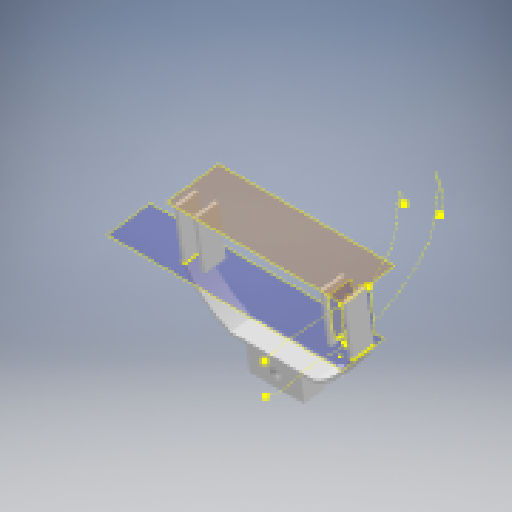
# Autodesk Inventor part: imu_mount
Saved by Autodesk Inventor 2024 (Build 280153000, 153)
## iProperties
Created: 2025-01-05
Part Number: imu_mount
Material: Generic
Document SubType Name: Modeling
Designer: Alex
Density: 1 g/cm^3
Appearance: Default
Author: Alex
Autodesk Inventor part; units mm, degrees
ref_plane "YZ Plane" through (0, 0, 0) normal (1, 0, 0) x (0, 1, 0)
ref_plane "XZ Plane" through (0, 0, 0) normal (0, 1, 0) x (-1, 0, 0)
ref_plane "XY Plane" through (0, 0, 0) normal (0, 0, 1) x (1, 0, 0)
sketch "Sketch1" plane through (0, 0, 0) normal (1, 0, 0) x (0, 1, 0)
  spline S0 degree 3 poles (-12.7596, 69.1102) (-15.2298, 61.5354) (-16.003, 54.7493) (-14.7341, 46.512) (-13.9585, 44.5403) (-12.6997, 40.1512) (-11.8689, 37.886) (-10.5675, 32.6221) (-10.0341, 29.5076) (-9.2498, 23.4956) (-9.1586, 20.4828) (-8.7362, 14.9457) (-8.298, 12.4468) (-8.4378, 7.0305) (-9.5013, 4.1287) (-9.4732, -0.7666) (-9.0812, -2.8089) (-8.7088, -6.0813) (-8.5625, -7.3217) (-8.4075, -8.5547) knots 0 0 0 0 0.241973 0.241973 0.332352 0.332352 0.424089 0.424089 0.541798 0.541798 0.658072 0.658072 0.76087 0.76087 0.872069 0.872069 0.951758 0.951758 1 1 1 1 construction
  spline S1 degree 3 poles (-8.4075, -8.5547) (-8.309, -9.3389) (-8.207, -10.12) (-7.7153, -13.7099) (-7.2118, -16.3393) (-6.3841, -22.1405) (-6.6665, -24.8142) (-5.6218, -28.3135) knots 0 0 0 0 0.119502 0.119502 0.553846 0.553846 1 1 1 1 construction
  spline S2 degree 3 poles (-5.6218, -28.3135) (-4.1228, -33.3346) (0.624, -41.8906) (3.9625, -48.268) (4.5736, -49.3774) (8.1498, -55.2575) (12.792, -61.9002) (17.7565, -68.8098) (19.0389, -70.9296) (26.2047, -78.6536) (35.4784, -85.2147) (49.0059, -92.3069) (55.6073, -92.3063) (68.5377, -94.6562) (74.996, -95.2419) (83.2666, -94.7145) (86.6124, -93.0362) (89.415, -93.015) (89.4684, -93.7995) (89.9841, -94.339) (90.2258, -94.7218) (89.67, -94.6644) (89.4356, -94.0936) (87.2104, -94.21) (84.8902, -94.7513) (80.0382, -96.05) (76.8909, -97.5474) (70.3825, -98.6246) (66.2945, -98.5443) (60.1257, -98.0168) (58.2481, -97.7121) (54.5132, -96.7744) (53.8418, -96.5978) (53.124, -96.4018) knots 0 0 0 0 0.060463 0.060463 0.088876 0.088876 0.149034 0.149034 0.189187 0.189187 0.280144 0.280144 0.381032 0.381032 0.501928 0.501928 0.587779 0.587779 0.653298 0.653298 0.710459 0.710459 0.757232 0.757232 0.814775 0.814775 0.872532 0.872532 0.939307 0.939307 0.990036 0.990036 1 1 1 1 construction
  spline S3 degree 3 poles (29.4725, -27.9505) (29.7232, -28.7604) (30.1347, -29.057) (32.5515, -32.3248) (34.3621, -34.4691) (37.878, -38.892) (37.7974, -39.3941) (41.586, -43.4308) (43.873, -45.7682) (49.5626, -50.6314) (51.8392, -50.9545) (60.2395, -53.9595) (66.6243, -55.2783) (76.7213, -57.0347) (82.4961, -56.8836) (87.4768, -57.2216) (87.6182, -57.0776) (89.8132, -57.4611) (91.5195, -57.7058) (92.188, -58.3474) (92.2546, -58.677) (90.5785, -59.545) (88.9174, -60.1439) (85.9397, -61.0379) (84.1283, -61.4382) (81.4338, -61.8751) (80.6089, -61.9837) (79.7567, -62.0753) knots 0 0 0 0 0.04737 0.04737 0.082065 0.082065 0.155524 0.155524 0.204555 0.204555 0.315622 0.315622 0.438816 0.438816 0.586443 0.586443 0.691275 0.691275 0.771281 0.771281 0.841079 0.841079 0.898194 0.898194 0.96846 0.96846 1 1 1 1 construction
  spline S4 degree 3 poles (28.8564, -23.7777) (28.9042, -24.5022) (28.9667, -25.1696) (29.2425, -26.8854) (29.3324, -27.498) (29.4725, -27.9505) knots 0 0 0 0 0.335914 0.335914 1 1 1 1 construction
  spline S5 degree 3 poles (27.5568, -11.1594) (27.8944, -13.1016) (28.2256, -15.1008) (28.7027, -19.1945) (28.7203, -21.7171) (28.8564, -23.7777) knots 0 0 0 0 0.46171 0.46171 1 1 1 1 construction
  spline S6 degree 3 poles (26.2925, -4.4074) (26.5211, -5.6352) (26.805, -6.8301) (27.1945, -9.1012) (27.3765, -10.1222) (27.5568, -11.1594) knots 0 0 0 0 0.568778 0.568778 1 1 1 1 construction
  spline S7 degree 3 poles (16.0432, 69.6268) (18.6865, 66.183) (20.6385, 61.0286) (22.3448, 51.7367) (22.7474, 48.7933) (23.2098, 43.6518) (23.1117, 41.1975) (23.483, 35.6031) (24.0275, 32.6396) (24.3977, 26.501) (24.1107, 23.3997) (24.6444, 17.6215) (25.4306, 14.8381) (25.926, 9.3729) (25.7134, 6.8435) (25.8358, 1.9262) (25.7789, -0.3383) (26.0611, -3.0685) (26.1687, -3.7428) (26.2925, -4.4074) knots 0 0 0 0 0.257427 0.257427 0.348427 0.348427 0.440796 0.440796 0.559313 0.559313 0.676387 0.676387 0.779892 0.779892 0.891856 0.891856 0.972092 0.972092 1 1 1 1 construction
  point P0 (0, 0)
ref_plane "Work Plane1" through (0, -5.6218, -28.3135) normal (-1, 0, 0) x (0, -0.1396054, 0.9902072)
ref_plane "Work Plane2" through (5.08, -5.6218, -28.3135) normal (-1, 0, 0) x (0, -0.1396054, 0.9902072)
sketch "Sketch2" plane through (5.08, -5.6218, -28.3135) normal (-1, 0, 0) x (0, -0.1396054, 0.9902072)
  line L0 (3.8114, -6.7133) -> (24.329, -6.7133)
  line L1 (24.329, -6.7133) -> (24.329, 43.4294)
  line L2 (24.329, 43.4294) -> (3.8114, 43.4294)
  line L3 (3.8114, 43.4294) -> (3.8114, -6.7133)
  point P0 (27.2514, 9.5195)
  constraints: 8 end point, 2 parallel, 1 horizontal, 1 perpendicular
extrude "Extrusion1" add sketch "Sketch2" against normal blind 3.175
ref_plane "Work Plane3" through (-11.938, -5.6218, -28.3135) normal (-1, 0, 0) x (0, -0.1396054, 0.9902072)
sketch "Sketch3" plane through (-11.938, -5.6218, -28.3135) normal (-1, 0, 0) x (0, -0.1396054, 0.9902072)
  line L0 (24.329, -6.7133) -> (24.329, 43.4294) projected
  line L1 (24.329, 43.4294) -> (3.8114, 43.4294) projected
  line L2 (3.8114, 43.4294) -> (3.8114, -6.7133) projected
  line L3 (3.8114, -6.7133) -> (24.329, -6.7133) projected
  point P0 (27.2514, 9.5195)
extrude "Extrusion2" add sketch "Sketch3" along normal blind 3.175
sketch "Sketch4" plane through (5.08, -5.6218, -28.3135) normal (-1, 0, 0) x (0, -0.1396054, 0.9902072)
  point P0 (27.2514, 9.5195)
ref_plane "Work Plane4" through (6.6675, 33.9858, 1.8402) normal (0, 0.9902072, 0.1396054) x (0, 0.1396054, -0.9902072)
ref_plane "Work Plane5" through (8.255, -12.8015, -25.4766) normal (0, -0.9902072, -0.1396054) x (0, -0.1396054, 0.9902072)
sketch "Sketch5" plane through (8.255, -12.8015, -25.4766) normal (0, -0.9902072, -0.1396054) x (0, -0.1396054, 0.9902072)
  line L0 (0, 20.193) -> (0, 23.368) construction
  line L1 (20.5176, 20.193) -> (20.5176, 23.368) construction
  line L2 (0, 23.368) -> (0, 209.8691) construction
  line L3 (0, 143.7138) -> (20.5176, 143.7138)
  line L4 (20.5176, 143.7138) -> (20.5176, 140.5388)
  line L5 (20.5176, 140.5388) -> (0, 140.5388)
  line L6 (0, 140.5388) -> (0, 143.7138)
  line L7 (0, 162.2606) -> (20.5176, 162.2606)
  line L8 (20.5176, 162.2606) -> (20.5176, 159.0856)
  line L9 (20.5176, 159.0856) -> (0, 159.0856)
  line L10 (0, 159.0856) -> (0, 162.2606)
  point P0 (23.44, 8.255)
  dimension "d6" = 3.175
  dimension "d7" = 3.175
  constraints: 18 end point, 4 parallel, 3 point on line, 2 horizontal, 2 perpendicular, 1 vertical
  measures "d6" distance of L3.end L4.end
  measures "d7" distance of L7.end L8.end
extrude "Extrusion3" add sketch "Sketch5" against normal up to surface (50.1427 mm away)
sketch "Sketch7" plane through (8.255, -12.8015, -25.4766) normal (0, -0.9902072, -0.1396054) x (0, -0.1396054, 0.9902072)
  line L0 (0, 3.175) -> (20.5176, 3.175) projected
  line L1 (0, 3.175) -> (0, 0) projected
  line L2 (20.5176, 0) -> (0, 0) projected
  line L3 (20.5176, 3.175) -> (20.5176, 0) projected
  line L4 (0, 159.0856) -> (20.5176, 159.0856) projected
  line L5 (20.5176, 159.0856) -> (20.5176, 162.2606) projected
  line L6 (20.5176, 162.2606) -> (0, 162.2606) projected
  line L7 (0, 162.2606) -> (0, 159.0856) projected
  point P0 (23.44, 8.255)
sketch "Sketch8" plane through (-154.0056, -15.6658, -5.16) normal (0, -0.1396054, 0.9902072) x (1, 0, 0)
  line L0 (159.0856, 0) -> (159.0856, 50.1427) projected
  line L1 (159.0856, 0) -> (162.2606, 0) projected
  line L2 (162.2606, 50.1427) -> (162.2606, 0) projected
  line L3 (159.0856, 50.1427) -> (162.2606, 50.1427) projected
  line L4 (3.175, 50.1427) -> (0, 50.1427) projected
  line L5 (0, 0) -> (0, 50.1427) projected
  line L6 (3.175, 0) -> (0, 0) projected
  line L7 (3.175, 0) -> (3.175, 50.1427) projected
  line L8 (120.8571, -41.0775) -> (41.4035, -41.0775)
  arc A0 (3.175, 0) -> (41.4035, -41.0775) centre (81.1303, 34.2212) ccw
  arc A1 (120.8571, -41.0775) -> (159.0856, 0) centre (81.1303, 34.2212) ccw
  arc A2 (121.0688, -44.2525) -> (162.2606, 0) centre (81.1303, 34.2212) ccw
  line L9 (121.0688, -44.2525) -> (41.1917, -44.2525)
  arc A3 (0, 0) -> (41.1917, -44.2525) centre (81.1303, 34.2212) ccw
  line L10 (0, 0) -> (0, 50.1427) projected
  line L11 (162.2606, 50.1427) -> (162.2606, 0) projected
  line L12 (200.1965, 0) -> (-37.9359, 0) projected
  point P0 (154.0056, 16.2328)
  dimension "d10" = 41.0775
  dimension "d12" = 3.175
  constraints: 8 point on circle, 4 centre point, 4 concentric, 4 end point, 2 horizontal
  measures "d10" distance between parallel lines of L12 L8
  measures "d12" distance between parallel lines of L8 L9
extrude "Extrusion4" add sketch "Sketch8" against normal up to surface (20.5176 mm away) contours L1 A2 L9 A3 L6 A0 L8 A1
sketch "Sketch9" plane through (-112.8138, -59.485, -11.3379) normal (0, -0.9902072, -0.1396054) x (1, 0, 0)
  line L0 (0, -20.5176) -> (79.8771, -20.5176) projected
  line L1 (79.8771, 0) -> (79.8771, -20.5176) projected
  line L2 (0, 0) -> (79.8771, 0) projected
  line L3 (0, 0) -> (0, -20.5176) projected
  line L4 (14.2872, 0) -> (65.5899, 0)
  line L5 (65.5899, 0) -> (65.5899, -20.5176)
  line L6 (65.5899, -20.5176) -> (14.2872, -20.5176)
  line L7 (14.2872, -20.5176) -> (14.2872, 0)
  point P0 (112.8138, 2.9224)
  point P1 (14.2872, -10.2588)
  point P2 (0, -10.2588)
  point P3 (79.8771, -10.2588)
  point P4 (65.5899, -10.2588)
  dimension "d15" = 14.2872
  dimension "d16" = 14.2872
  constraints: 8 end point, 4 midpoint, 2 parallel, 2 point on line, 1 horizontal, 1 perpendicular
  measures "d15" distance of point (14.287, -10.259) point (0, -10.259)
  measures "d16" distance of point (79.877, -10.259) point (65.59, -10.259)
extrude "Extrusion5" add sketch "Sketch9" along normal blind 25.4 contours L7 L2 L5 L0
sketch "Sketch10" plane through (-112.6021, -56.3411, -10.8946) normal (0, -0.1396054, 0.9902072) x (1, 0, 0)
  line L0 (65.3781, -28.575) -> (14.0755, -28.575) projected
  line L1 (-0.2118, -3.175) -> (14.0755, -3.175) projected
  line L2 (65.3781, -28.575) -> (14.0755, -28.575)
  line L3 (14.0755, -28.575) -> (14.0755, -3.175)
  line L4 (14.0755, -3.175) -> (65.3781, -3.175)
  line L5 (65.3781, -3.175) -> (65.3781, -28.575)
  circle A0 centre (39.7268, -15.875) radius 5
  point P0 (112.6021, 57.3103)
  dimension "d19" = 10
  constraints: 8 end point, 2 parallel, 1 centre point, 1 horizontal, 1 perpendicular
  measures "d19" diameter of A0
hole "Hole1" at (-72.8753, -72.0607, -13.1109) direction (0, 0.1396054, -0.9902072) diameter 8.647 end through all thread size "M10x1.25" class "6H" standard "ANSI Metric M Profile"
sketch "Sketch11" plane through (-112.6021, -56.3411, -10.8946) normal (0, -0.1396054, 0.9902072) x (1, 0, 0)
  point P0 (112.6021, 57.3103)
equation "\"d16\" = d15"
body "Solid1"
